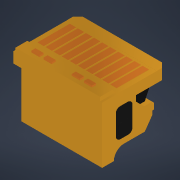
# Autodesk Inventor part: McCrea_roof_walle
Saved by Autodesk Inventor 2022 (Build 260153000, 153)
## iProperties
Created: 2022-02-04
Part Number: McCrea_roof_walle
Material: Generic
Document SubType Name: Modeling
Designer: MatusBarany
Density: 1 g/cm^3
Appearance: Metal 1800F Hot
Author: MatusBarany
Autodesk Inventor part; units mm, degrees
ref_plane "YZ Plane" through (0, 0, 0) normal (1, 0, 0) x (0, 1, 0)
ref_plane "XZ Plane" through (0, 0, 0) normal (0, 1, 0) x (-1, 0, 0)
sketch "Sketch1" plane through (0, 0, 0) normal (0, 0, 1) x (1, 0, 0)
  line L0 (-554.5833, 364.6296) -> (545.4167, 364.6296)
  line L1 (545.4167, 364.6296) -> (545.4167, 214.6296)
  line L2 (545.4167, 214.6296) -> (-554.5833, 214.6296)
  line L3 (-554.5833, 214.6296) -> (-554.5833, 364.6296)
  point P0 (0, 0)
  dimension "d0" = 1100
  dimension "d1" = 150
  constraints: 8 end point, 2 parallel, 1 horizontal, 1 perpendicular
  measures "d0" distance of L0.start L0.end
  measures "d1" distance of L0.end L1.end
extrude "Extrusion1" add sketch "Sketch1" along normal blind 800
sketch "Sketch2" plane through (-554.5833, 214.6296, 0) normal (0, -1, 0) x (1, 0, 0)
  line L0 (0, 0) -> (1100, 0) projected
  line L1 (1100, 0) -> (1100, 800) projected
  line L2 (0, 800) -> (1100, 800) projected
  line L3 (0, 0) -> (0, 800) projected
  line L4 (1050, 750) -> (50, 750)
  line L5 (50, 750) -> (50, 130)
  line L6 (50, 130) -> (1050, 130)
  line L7 (1050, 130) -> (1050, 750)
  line L8 (550, 750) -> (550, 130) construction
  point P0 (554.5833, 0)
  dimension "d4" = 130
  dimension "d5" = 50
  dimension "d8" = 1000
  dimension "d9" = 1100
  dimension "d12" = 550
  constraints: 10 end point, 2 midpoint, 2 parallel, 1 horizontal, 1 perpendicular
  measures "d4" distance between parallel lines of L0 L6
  measures "d5" distance between parallel lines of L4 L2
  measures "d8" distance of L4.start L4.end
  measures "d9" distance of L2.start L1.end
  measures "d12" distance between parallel lines of L3 L8
extrude "Extrusion2" add sketch "Sketch2" along normal blind 600 contours L7 L6 L5 L4
sketch "Sketch3" plane through (495.4167, 214.6296, 750) normal (1, 0, 0) x (0, 0, -1)
  line L0 (0, 0) -> (620, 0) projected
  line L1 (0, 0) -> (0, -600) projected
  line L2 (620, -600) -> (0, -600) projected
  line L3 (620, 0) -> (620, -600) projected
  line L4 (0, -600) -> (620, -600) projected
  arc A0 (270, -475) -> (145, -600) centre (270, -600) ccw
  line L5 (270, -475) -> (620, -475)
  line L6 (620, 0) -> (620, -600) projected
  line L7 (620, -600) -> (0, -600) projected
  point P0 (750, -214.6296)
  dimension "d15" = 250
  dimension "d16" = 350
  constraints: 3 point on line, 2 end point, 2 point on circle, 1 centre point, 1 horizontal, 1 parallel, 1 tangent
  measures "d15" diameter of A0
  measures "d16" distance of L5.start L5.end
extrude "Extrusion3" cut sketch "Sketch3" against normal through all contours L3 L2 A0 L5
sketch "Sketch4" plane through (495.4167, 214.6296, 750) normal (1, 0, 0) x (0, 0, -1)
  line L0 (620, 0) -> (420, 0)
  line L1 (420, 0) -> (420, -100)
  line L2 (520, -200) -> (620, -200)
  line L3 (620, -200) -> (620, 0)
  line L4 (420, -100) -> (520, -200)
  point P0 (750, -214.6296)
  point P1 (420, -200)
  dimension "d19" = 200
  dimension "d20" = 200
  dimension "d21" = 100
  dimension "d22" = 100
  constraints: 10 end point, 2 parallel, 2 point on line, 1 horizontal, 1 perpendicular
  measures "d19" distance of point (420, -200) L2.end
  measures "d20" distance of L0.end point (420, -200)
  measures "d21" distance of L1.end point (420, -200)
  measures "d22" distance of L2.start point (420, -200)
extrude "Extrusion4" cut sketch "Sketch4" against normal through all
sketch "Sketch5" plane through (-554.5833, 214.6296, 0) normal (0, -1, 0) x (1, 0, 0)
  line L0 (1100, 0) -> (0, 0) projected
  line L1 (0, 0) -> (0, 800) projected
  line L2 (1100, 800) -> (0, 800) projected
  line L3 (1100, 0) -> (1100, 800) projected
  line L4 (1000, 80) -> (100, 80)
  line L5 (100, 80) -> (100, 330)
  line L6 (100, 330) -> (1000, 330)
  line L7 (1000, 330) -> (1000, 80)
  point P0 (554.5833, 0)
  dimension "d25" = 900
  dimension "d26" = 250
  dimension "d27" = 80
  dimension "d28" = 100
  constraints: 8 end point, 2 parallel, 1 horizontal, 1 perpendicular
  measures "d25" distance between parallel lines of L5 L7
  measures "d26" distance between parallel lines of L4 L6
  measures "d27" distance between parallel lines of L0 L4
  measures "d28" distance between parallel lines of L1 L5
extrude "Extrusion5" add sketch "Sketch5" along normal blind 200 contours L4 L5 L6 L7
sketch "Sketch7" plane through (-454.5833, 214.6296, 80) normal (-1, 0, 0) x (0, 0, 1)
  line L0 (250, -100) -> (150, -200) projected
  line L1 (250, 0) -> (250, -100) projected
  line L2 (0, 0) -> (250, 0) projected
  line L3 (0, 0) -> (0, -200) projected
  line L4 (50, -200) -> (0, -200) projected
  line L5 (150, -200) -> (50, -200) projected
  line L6 (0, 0) -> (91.6515, -200)
  line L7 (50, -200) -> (150, -200) projected
  point P0 (-80, -214.6296)
  point P1 (91.6515, -200)
  dimension "d35" = 220
  constraints: 2 end point, 1 point on line
  measures "d35" distance of L2.start L6.end
extrude "Extrusion6" cut sketch "Sketch7" against normal through all contours L5 L4 L3 L6
sketch "Sketch8" plane through (445.4167, 14.6296, 171.6515) normal (0, -0.4165978, -0.9090909) x (-1, 0, 0)
  line L0 (0, 0) -> (0, 220) projected
  line L1 (900, 0) -> (0, 0) projected
  line L2 (900, 220) -> (900, 0) projected
  line L3 (0, 220) -> (900, 220) projected
  line L4 (0, 220) -> (900, 220) projected
  line L5 (450, 220) -> (450, 17.3519)
  line L6 (950, 17.3519) -> (-50, 17.3519) projected
  line L7 (292.5, 220) -> (332.5, 220)
  line L8 (332.5, 220) -> (332.5, 17.3519)
  line L9 (332.5, 17.3519) -> (292.5, 17.3519)
  line L10 (292.5, 17.3519) -> (292.5, 220)
  line L11 (257.5, 220) -> (292.5, 220)
  line L12 (292.5, 220) -> (292.5, 190)
  line L13 (292.5, 190) -> (257.5, 190)
  line L14 (257.5, 190) -> (257.5, 220)
  line L15 (607.5, 220) -> (567.5, 220)
  line L16 (567.5, 220) -> (567.5, 17.3519)
  line L17 (567.5, 17.3519) -> (607.5, 17.3519)
  line L18 (607.5, 17.3519) -> (607.5, 220)
  line L19 (642.5, 220) -> (607.5, 220)
  line L20 (607.5, 190) -> (642.5, 190)
  line L21 (642.5, 190) -> (642.5, 220)
  point P0 (445.4167, 58.21)
  point P1 (292.5, 17.3519)
  point P2 (567.5, 220)
  point P3 (567.5, 17.3519)
  point P4 (607.5, 17.3519)
  point P5 (642.5, 220)
  dimension "d38" = 40
  dimension "d39" = 75
  dimension "d40" = 235
  dimension "d41" = 30
  constraints: 32 end point, 8 symmetric about line, 5 point on line, 4 parallel, 2 horizontal, 2 midpoint, 2 perpendicular
  measures "d38" distance between parallel lines of L8 L10
  measures "d39" distance between parallel lines of L8 L14
  measures "d40" diameter of L8 L5
  measures "d41" distance of L13.end L11.start
extrude "Extrusion7" add sketch "Sketch8" along normal blind 10 contours L10 L3 L8 L6 | L3 L10 L13 L14 | L6 L16 L3 L18 | L21 L20 L18 L3
sketch "Sketch9" plane through (495.4167, 14.6296, 230) normal (0, 1, 0) x (1, 0, 0)
  line L0 (-950, 58.3485) -> (-50, 58.3485) projected
  line L1 (-50, 58.3485) -> (-50, 0) projected
  line L2 (0, 0) -> (-50, 0) projected
  line L3 (0, 100) -> (0, 0) projected
  line L4 (-1000, 100) -> (0, 100) projected
  line L5 (-1000, 0) -> (-1000, 100) projected
  line L6 (-950, 0) -> (-1000, 0) projected
  line L7 (-950, 0) -> (-950, 58.3485) projected
  line L8 (-950, 58.3485) -> (-50, 58.3485) projected
  line L9 (-75, 58.3485) -> (-925, 58.3485)
  line L10 (-925, 58.3485) -> (-925, 83.3485)
  line L11 (-925, 83.3485) -> (-75, 83.3485)
  line L12 (-75, 83.3485) -> (-75, 58.3485)
  point P0 (-495.4167, 230)
  point P1 (-925, 58.3485)
  dimension "d44" = 900
  dimension "d45" = 850
  dimension "d46" = 25
  dimension "d47" = 25
  constraints: 8 end point, 2 parallel, 1 horizontal, 1 perpendicular, 1 point on line
  measures "d44" distance of L0.start L0.end
  measures "d45" distance of L10.end L11.end
  measures "d46" distance between parallel lines of L7 L10
  measures "d47" distance between parallel lines of L0 L11
extrude "Extrusion8" add sketch "Sketch9" along normal blind 10 contours L10 L11 L12 L0
ref_plane "Work Plane1" through (-4.5833, -385.3704, 750) normal (-1, 0, 0) x (0, 0, 1)
sketch "Sketch10" plane through (495.4167, -260.3704, 130) normal (0, 0, -1) x (-1, 0, 0)
  line L0 (0, 475) -> (0, -125) projected
  line L1 (0, 255) -> (160, 255)
  line L2 (160, 255) -> (160, 180)
  line L3 (160, 180) -> (0, 180)
  line L4 (0, 180) -> (0, 255)
  line L5 (1000, 275) -> (0, 275) projected
  point P0 (495.4167, 260.3704)
  point P1 (0, 180)
  dimension "d50" = 75
  dimension "d51" = 160
  dimension "d52" = 20
  constraints: 8 end point, 2 parallel, 1 horizontal, 1 perpendicular, 1 point on line
  measures "d50" distance between parallel lines of L1 L3
  measures "d51" distance between parallel lines of L0 L2
  measures "d52" distance between parallel lines of L5 L1
extrude "Extrusion9" add sketch "Sketch10" along normal blind 20
sketch "Sketch11" plane through (495.4167, -260.3704, 110) normal (0, 0, -1) x (-1, 0, 0)
  line L0 (160, 255) -> (0, 255) projected
  line L1 (0, 255) -> (0, 180) projected
  line L2 (0, 180) -> (160, 180) projected
  line L3 (160, 180) -> (160, 255) projected
  circle A0 centre (37.5, 217.5) radius 37.5
  circle A1 centre (122.5, 217.5) radius 37.5
  line L4 (160, 180) -> (160, 255) projected
  line L5 (160, 255) -> (0, 255) projected
  line L6 (0, 180) -> (160, 180) projected
  circle A2 centre (37.5, 217.5) radius 22.5
  circle A3 centre (122.5, 217.5) radius 22.5
  point P0 (495.4167, 260.3704)
  dimension "d55" = 45
  dimension "d56" = 45
  constraints: 6 tangent, 4 centre point
  measures "d55" diameter of A3
  measures "d56" diameter of A2
extrude "Extrusion10" cut sketch "Sketch11" against normal blind 5 contours A2 | A3
sketch "Sketch13" plane through (495.4167, -385.3704, 750) normal (1, 0, 0) x (0, 0, -1)
  line L0 (220, 550) -> (320, 550)
  line L1 (370, 500) -> (370, 250)
  line L2 (320, 200) -> (220, 200)
  line L3 (170, 250) -> (170, 500)
  line L4 (420, 500) -> (420, 600) projected
  line L5 (750, 600) -> (-50, 600) projected
  arc A0 (370, 500) -> (320, 550) centre (320, 500) ccw
  arc A1 (220, 550) -> (170, 500) centre (220, 500) ccw
  arc A2 (170, 250) -> (220, 200) centre (220, 250) ccw
  arc A3 (320, 200) -> (370, 250) centre (320, 250) ccw
  point P0 (750, 385.3704)
  point P1 (370, 200)
  point P2 (370, 550)
  dimension "d59" = 200
  dimension "d60" = 350
  dimension "d61" = 50
  dimension "d62" = 50
  dimension "d68" = 50
  constraints: 8 end point, 8 point on circle, 8 tangent, 4 centre point, 4 point on line, 3 equal radius, 2 parallel, 1 horizontal, 1 perpendicular
  measures "d59" distance between parallel lines of L1 L3
  measures "d60" distance of point (370, 550) point (370, 200)
  measures "d61" distance between parallel lines of L4 L1
  measures "d62" distance between parallel lines of L5 L0
  measures "d68" radius of A0
sketch "Sketch14" plane through (495.4167, -385.3704, 750) normal (1, 0, 0) x (0, 0, -1)
  line L0 (270, 125) -> (620, 125) projected
  line L1 (528.2278, 125) -> (620, 256.0643)
  line L2 (620, 305) -> (620, 125) projected
  point P0 (750, 385.3704)
  dimension "d64" = 35
  dimension "d65" = 160
  constraints: 2 end point, 2 point on line
  measures "d64" angle of L2 L1
  measures "d65" distance of L1.start L1.end
extrude "Extrusion11" cut sketch "Sketch14" against normal through all
extrude "Extrusion12" add sketch "Sketch13" along normal blind 5
sketch "Sketch15" plane through (500.4167, -385.3704, 750) normal (1, 0, 0) x (0, 0, -1)
  line L0 (220, 200) -> (320, 200) projected
  arc A0 (320, 200) -> (370, 250) centre (320, 250) ccw projected
  line L1 (370, 250) -> (370, 500) projected
  arc A1 (370, 500) -> (320, 550) centre (320, 500) ccw projected
  line L2 (320, 550) -> (220, 550) projected
  arc A2 (220, 550) -> (170, 500) centre (220, 500) ccw projected
  line L3 (170, 500) -> (170, 250) projected
  arc A3 (170, 250) -> (220, 200) centre (220, 250) ccw projected
  line L4 (240, 380) -> (300, 380)
  line L5 (350, 330) -> (350, 270)
  line L6 (300, 220) -> (240, 220)
  line L7 (190, 270) -> (190, 330)
  arc A4 (190, 270) -> (240, 220) centre (240, 270) ccw
  arc A5 (240, 380) -> (190, 330) centre (240, 330) ccw
  arc A6 (350, 330) -> (300, 380) centre (300, 330) ccw
  arc A7 (300, 220) -> (350, 270) centre (300, 270) ccw
  point P0 (750, 385.3704)
  dimension "d72" = 50
  dimension "d73" = 160
  dimension "d74" = 20
  dimension "d75" = 20
  dimension "d76" = 160
  constraints: 8 end point, 8 point on circle, 8 tangent, 4 centre point, 3 equal radius, 2 parallel, 1 horizontal, 1 perpendicular
  measures "d72" radius of A4
  measures "d73" distance between parallel lines of L5 L7
  measures "d74" distance between parallel lines of L3 L7
  measures "d75" distance between parallel lines of L0 L6
  measures "d76" distance between parallel lines of L4 L6
extrude "Extrusion13" add sketch "Sketch15" along normal blind 5 contours L4 A6 L5 A7 L6 A4 L7 A5
sketch "Sketch16" plane through (-554.5833, 364.6296, 0) normal (0, 1, 0) x (1, 0, 0)
  line L0 (25, -800) -> (1075, -800)
  line L1 (1075, -800) -> (1075, -600)
  line L2 (1075, -600) -> (25, -600)
  line L3 (25, -600) -> (25, -800)
  line L4 (1100, -800) -> (0, -800) projected
  line L5 (0, 0) -> (0, -800) projected
  point P0 (554.5833, 0)
  dimension "d79" = 1050
  dimension "d80" = 25
  dimension "d81" = 200
  constraints: 8 end point, 2 parallel, 1 collinear, 1 horizontal, 1 perpendicular
  measures "d79" distance of L1.end L2.end
  measures "d80" distance between parallel lines of L5 L3
  measures "d81" distance between parallel lines of L0 L2
extrude "Extrusion14" add sketch "Sketch16" along normal blind 50
chamfer "Chamfer1" distance 50 angle 45 1 edges at (-4.5833, 414.6296, 600)
sketch "Sketch17" plane through (-554.5833, 414.6296, 0) normal (0, 1, 0) x (1, 0, 0)
  line L0 (50, -750) -> (1050, -750) projected
  line L1 (925, -750) -> (825, -750)
  line L2 (825, -750) -> (825, -700)
  line L3 (825, -700) -> (925, -700)
  line L4 (925, -700) -> (925, -750)
  line L5 (775, -750) -> (675, -750)
  line L6 (675, -750) -> (675, -700)
  line L7 (675, -700) -> (775, -700)
  line L8 (775, -700) -> (775, -750)
  line L9 (1075, -800) -> (1075, -650) projected
  point P0 (554.5833, 0)
  point P1 (675, -750)
  dimension "d87" = 100
  dimension "d88" = 100
  dimension "d89" = 50
  dimension "d90" = 50
  dimension "d91" = 50
  dimension "d92" = 150
  constraints: 16 end point, 4 parallel, 3 point on line, 2 horizontal, 2 perpendicular
  measures "d87" distance between parallel lines of L2 L4
  measures "d88" distance between parallel lines of L6 L8
  measures "d89" distance between parallel lines of L3 L0
  measures "d90" distance between parallel lines of L7 L0
  measures "d91" distance between parallel lines of L8 L2
  measures "d92" distance between parallel lines of L4 L9
extrude "Extrusion15" add sketch "Sketch17" along normal blind 20
sketch "Sketch18" plane through (495.4167, 14.6296, 130) normal (0, 0, -1) x (-1, 0, 0)
  line L0 (410, -65) -> (590, -65) construction
  line L1 (410, -80) -> (590, -80)
  line L2 (590, -50) -> (410, -50)
  arc A0 (410, -50) -> (410, -80) centre (410, -65) ccw
  arc A1 (590, -80) -> (590, -50) centre (590, -65) ccw
  line L3 (1000, 0) -> (1000, -143.9357) projected
  line L4 (1000, 0) -> (0, 0) projected
  point P0 (495.4167, -14.6296)
  point P1 (500, -65)
  dimension "d95" = 500
  dimension "d96" = 30
  dimension "d97" = 50
  dimension "d98" = 180
  constraints: 8 end point, 4 point on circle, 4 tangent, 2 centre point, 1 horizontal, 1 midpoint, 1 parallel
  measures "d95" distance from line of L3 point (500, -65)
  measures "d96" distance between parallel lines of L2 L1
  measures "d97" distance between parallel lines of L4 L2
  measures "d98" distance of L0.end L0.start
extrude "Extrusion16" add sketch "Sketch18" along normal blind 5
mirror "Mirror1" about plane through (-4.5833, -385.3704, 750) normal (-1, 0, 0) of "Extrusion10", "Extrusion9"
mirror "Mirror2" about plane through (-4.5833, -385.3704, 750) normal (-1, 0, 0) of "Extrusion15"
mirror "Mirror3" about plane through (-4.5833, -385.3704, 750) normal (-1, 0, 0) of "Extrusion13", "Extrusion12"
sketch "Sketch19" plane through (495.4167, -129.306, 130) normal (0, -0.5735764, -0.819152) x (-1, 0, 0)
  line L0 (1000, 0) -> (1000, -160) projected
  line L1 (0, 0) -> (1000, 0) projected
  line L2 (0, -160) -> (0, 0) projected
  line L3 (1000, -160) -> (0, -160) projected
  line L4 (0, 0) -> (1000, 0) projected
  line L5 (1000, -160) -> (0, -160) projected
  line L6 (375, 0) -> (625, 0)
  line L7 (625, 0) -> (625, -160)
  line L8 (625, -160) -> (375, -160)
  line L9 (375, -160) -> (375, 0)
  line L10 (375, -135) -> (625, -135)
  line L11 (500, 0) -> (500, -135)
  point P0 (495.4167, 180.4862)
  point P1 (625, 0)
  point P2 (375, 0)
  dimension "d101" = 250
  dimension "d102" = 500
  dimension "d103" = 135
  constraints: 12 end point, 4 point on line, 2 midpoint, 2 parallel, 2 perpendicular, 1 horizontal
  measures "d101" distance between parallel lines of L7 L9
  measures "d102" distance between parallel lines of L0 L11
  measures "d103" distance between parallel lines of L1 L10
extrude "Extrusion17" add sketch "Sketch19" along normal blind 10 contours L7 L10 L11 L1 | L11 L10 L9 L1
sketch "Sketch20" plane through (495.4167, 14.6296, 130) normal (0, 0, -1) x (-1, 0, 0)
  line L0 (840, -20) -> (1000, -20) projected
  line L1 (1000, 0) -> (1000, -20) projected
  line L2 (1000, 0) -> (0, 0) projected
  line L3 (0, 0) -> (0, -20) projected
  line L4 (0, -20) -> (160, -20) projected
  line L5 (160, -20) -> (160, -95) projected
  line L6 (160, -95) -> (0, -95) projected
  line L7 (0, -95) -> (0, -143.9357) projected
  line L8 (0, -143.9357) -> (375, -143.9357) projected
  line L9 (375, -143.9357) -> (625, -143.9357) projected
  line L10 (625, -143.9357) -> (1000, -143.9357) projected
  line L11 (1000, -95) -> (1000, -143.9357) projected
  line L12 (1000, -95) -> (840, -95) projected
  line L13 (840, -95) -> (840, -20) projected
  line L14 (590, -80) -> (410, -80) projected
  arc A0 (410, -50) -> (410, -80) centre (410, -65) ccw projected
  line L15 (410, -50) -> (590, -50) projected
  arc A1 (590, -80) -> (590, -50) centre (590, -65) ccw projected
  line L16 (625, -149.6714) -> (375, -149.6714) projected
  line L17 (375, -149.6714) -> (625, -149.6714)
  line L18 (625, -149.6714) -> (625, -99.6714)
  line L19 (625, -99.6714) -> (375, -99.6714)
  line L20 (375, -99.6714) -> (375, -149.6714)
  point P0 (495.4167, -14.6296)
  dimension "d106" = 250
  dimension "d107" = 250
  dimension "d108" = 50
  constraints: 8 end point, 2 parallel, 1 horizontal, 1 perpendicular
  measures "d106" distance of L16.start L16.end
  measures "d107" distance of L18.end L19.end
  measures "d108" distance between parallel lines of L19 L17
extrude "Extrusion18" add sketch "Sketch20" along normal blind 10 contours L9 L20 L19 L18
sketch "Sketch21" plane through (120.4167, -129.306, 130) normal (1, 0, 0) x (0, 0, -1)
  line L0 (0, 0) -> (0, 44.2642) projected
  line L1 (0, 0) -> (10, 0) projected
  line L2 (10, 44.2642) -> (10, 0) projected
  line L3 (0, 44.2642) -> (10, 44.2642) projected
  line L4 (-77.4328, -110.5855) -> (0, 0) projected
  line L5 (-77.4328, -110.5855) -> (-69.2413, -116.3213) projected
  line L6 (8.1915, -5.7358) -> (-69.2413, -116.3213) projected
  line L7 (0, 0) -> (8.1915, -5.7358) projected
  line L8 (0, 0) -> (8.1915, -5.7358) projected
  line L9 (10, 0) -> (8.1915, -5.7358)
  point P0 (130, 129.306)
  constraints: 2 end point
extrude "Extrusion19" add sketch "Sketch21" against normal blind 250 contours L1 L9 L7
sketch "Sketch22" plane through (495.4167, 14.6296, 120) normal (0, 0, -1) x (-1, 0, 0)
  line L0 (375, -99.6714) -> (375, -143.9357) projected
  line L1 (375, -143.9357) -> (625, -143.9357) projected
  line L2 (625, -143.9357) -> (625, -99.6714) projected
  line L3 (625, -99.6714) -> (375, -99.6714) projected
  line L4 (625, -260.257) -> (625, -149.6714) projected
  line L5 (625, -149.6714) -> (375, -149.6714) projected
  line L6 (375, -149.6714) -> (375, -260.257) projected
  line L7 (375, -260.257) -> (625, -260.257) projected
  line L8 (375, -149.6714) -> (375, -143.9357) projected
  line L9 (625, -149.6714) -> (375, -149.6714) projected
  line L10 (625, -143.9357) -> (625, -149.6714) projected
  line L11 (375, -143.9357) -> (625, -143.9357) projected
  line L12 (385, -104.6714) -> (615, -104.6714)
  line L13 (615, -104.6714) -> (615, -114.6714)
  line L14 (615, -114.6714) -> (385, -114.6714)
  line L15 (385, -114.6714) -> (385, -104.6714)
  point P0 (495.4167, -14.6296)
  dimension "d113" = 5
  dimension "d114" = 10
  dimension "d115" = 10
  dimension "d116" = 230
  constraints: 8 end point, 2 parallel, 1 horizontal, 1 perpendicular
  measures "d113" distance between parallel lines of L3 L12
  measures "d114" distance between parallel lines of L12 L14
  measures "d115" distance between parallel lines of L2 L13
  measures "d116" distance between parallel lines of L13 L15
extrude "Extrusion20" add sketch "Sketch22" along normal blind 5 contours L12 L13 L14 L15
pattern_linear "Rectangular Pattern1" count 3 spacing 15 along (0, -1, 0) of "Extrusion20"
sketch "Sketch23" plane through (495.4167, -135.0418, 121.8085) normal (0, -0.5735764, -0.819152) x (-1, 0, 0)
  line L0 (385, 1) -> (615, 1)
  line L1 (615, 1) -> (615, -9)
  line L2 (615, -9) -> (385, -9)
  line L3 (385, -9) -> (385, 1)
  line L4 (625, 0) -> (625, -135) projected
  line L5 (625, 0) -> (375, 0) projected
  point P0 (495.4167, 180.4862)
  dimension "d122" = 230
  dimension "d123" = 10
  dimension "d124" = 10
  dimension "d128" = 1
  constraints: 8 end point, 2 parallel, 1 horizontal, 1 perpendicular
  measures "d122" distance of L1.end L2.end
  measures "d123" distance of L0.end L1.end
  measures "d124" distance between parallel lines of L4 L1
  measures "d128" distance between parallel lines of L0 L5
extrude "Extrusion21" add sketch "Sketch23" along normal blind 5
pattern_linear "Rectangular Pattern2" count 9 spacing 15 along (0, -0.819152, 0.5735764) of "Extrusion21"
chamfer "Chamfer2" distance 3 angle 45 7 edges at (-4.5833, -85.0418, 120) (120.4167, -107.1739, 120) (-129.5833, -107.1739, 120) (-129.5833, -132.1739, 120.9042) (-129.5833, -190.3346, 160.5249) (-4.5833, -245.6273, 199.2413) (120.4167, -190.3346, 160.5249)
fillet "Fillet1" radius 2 2 edges at (480.4167, -42.8704, 110) (395.4167, -42.8704, 110)
fillet "Fillet2" radius 2 2 edges at (-404.5833, -42.8704, 110) (-489.5833, -42.8704, 110)
chamfer "Chamfer4" distance 60 angle 45 2 edges at (545.4167, 289.6296, 0) (-554.5833, 289.6296, 0)
chamfer "Chamfer5" distance 20 angle 45 7 edges at (545.4167, 214.6296, 70) (545.4167, 214.6296, 440) (515.4167, 214.6296, 30) (-4.5833, 214.6296, 0) (-524.5833, 214.6296, 30) (-554.5833, 214.6296, 430) (-4.5833, 214.6296, 800)
sketch "Sketch24" plane through (187.9167, 187.3569, 92.4979) normal (1, 0, 0) x (0, -0.4165978, -0.9090909)
  line L0 (0, 0) -> (0, 30) projected
  line L1 (0, 0) -> (10, 0) projected
  line L2 (10, 30) -> (10, 0) projected
  line L3 (0, 30) -> (10, 30) projected
  line L4 (-636.3636, -261.6185) -> (10.6507, 34.8807) projected
  line L5 (10.6507, 34.8807) -> (9.8499, 56.5138) projected
  line L6 (9.8499, 56.5138) -> (-662.8774, -251.7686) projected
  line L7 (-662.8774, -251.7686) -> (-636.3636, -261.6185) projected
  line L8 (10, 30) -> (10, 34.5826)
  point P0 (162.1415, -131.79)
  constraints: 2 end point, 1 point on line, 1 vertical
extrude "Extrusion22" add sketch "Sketch24" against normal blind 75 contours L4 L8 L3
sketch "Sketch25" plane through (-122.0833, 30.4041, 164.4227) normal (1, 0, 0) x (0, -0.4165978, -0.9090909)
  line L0 (0, 202.6481) -> (10, 202.6481) projected
  line L1 (10, 202.6481) -> (10, 207.2306)
  line L2 (10.6507, 207.5288) -> (-636.3636, -88.9704) projected
  point P0 (162.1415, 40.858)
  dimension "d148" = 4.5826
  constraints: 2 end point, 1 point on line, 1 vertical
  measures "d148" distance of L0.end L1.end
extrude "Extrusion23" add sketch "Sketch25" against normal blind 75
chamfer "Chamfer6" distance 5 angle 45 8 edges at (112.9167, 120.4339, 112.1659) (152.9167, 104.7145, 119.3694) (170.4167, 183.1909, 83.407) (187.9167, 198.9103, 76.2035) (-122.0833, 120.4339, 112.1659) (-179.5833, 183.1909, 83.407) (-162.0833, 104.7145, 119.3694) (-197.0833, 198.9103, 76.2035)
sketch "Sketch26" plane through (-529.5833, 364.6296, 600) normal (0, 1, 0) x (1, 0, 0)
  line L0 (-25, 540) -> (35, 600) projected
  line L1 (-25, 540) -> (-25, -200) projected
  line L2 (0, -200) -> (-25, -200) projected
  line L3 (0, -200) -> (0, 0) projected
  line L4 (0, 0) -> (1050, 0) projected
  line L5 (1050, 0) -> (1050, -200) projected
  line L6 (1075, -200) -> (1050, -200) projected
  line L7 (1075, 540) -> (1075, -200) projected
  line L8 (1015, 600) -> (1075, 540) projected
  line L9 (1015, 600) -> (35, 600) projected
  line L10 (-25, -200) -> (-25, 540) projected
  line L11 (-25, 475) -> (1075, 475)
  line L12 (1075, 540) -> (1075, -200) projected
  point P0 (529.5833, 600)
  point P1 (-25, 475)
  point P2 (1075, 475)
  dimension "d154" = 125
  constraints: 2 end point, 2 point on line, 1 perpendicular
  measures "d154" distance between parallel lines of L9 L11
extrude "Extrusion24" add sketch "Sketch26" along normal blind 1 contours L0 L9 L8 L7 L11 L1
sketch "Sketch27" plane through (-529.5833, 364.6296, 600) normal (0, 1, 0) x (1, 0, 0)
  line L0 (935, 40) -> (1015, 40)
  line L1 (1015, 40) -> (1015, 440)
  line L2 (1015, 440) -> (935, 440)
  line L3 (935, 440) -> (935, 40)
  line L4 (-25, 475) -> (1075, 475) projected
  line L5 (1075, 475) -> (1075, -200) projected
  point P0 (529.5833, 600)
  dimension "d157" = 80
  dimension "d158" = 400
  dimension "d159" = 35
  dimension "d160" = 60
  constraints: 8 end point, 2 parallel, 1 horizontal, 1 perpendicular
  measures "d157" distance between parallel lines of L3 L1
  measures "d158" distance between parallel lines of L0 L2
  measures "d159" distance between parallel lines of L4 L2
  measures "d160" distance between parallel lines of L1 L5
extrude "Extrusion25" add sketch "Sketch27" along normal blind 5
pattern_linear "Rectangular Pattern3" count 10 spacing 100 along (-1, 0, 0) of "Extrusion25"
equation "\"d12\" = 0.5 * d9"
equation "\"d22\" = d21"
equation "\"d56\" = d55"
equation "\"d76\" = d73"
equation "\"d107\" = d106"
body "Solid1"
